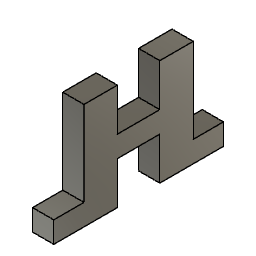
H shape (Autodesk Fusion 360 design; units mm, degrees)
Autodesk Fusion 360 part; units mm, degrees
sketch "Sketch1" plane through (0, 0, 0) normal (1, 0, 0) x (0, 1, 0)
  line L0 (0, -5.7569) -> (0, 10)
  line L1 (0, 10) -> (14.2431, 10)
  line L2 (14.2431, 10) -> (14.2431, 50)
  line L3 (14.2431, 50) -> (30, 50)
  line L4 (30, 30) -> (50, 30)
  line L5 (50, 30) -> (50, 50)
  line L6 (50, 50) -> (65.7569, 50)
  line L7 (25, -25) -> (23.7742, -25.0601)
  line L8 (65.7569, 50) -> (65.7569, 10)
  line L9 (65.7569, 10) -> (80, 10)
  line L10 (80, 10) -> (80, 0)
  line L11 (0, -5.7569) -> (0, 0)
  line L12 (30, 50) -> (30, 30)
  line L13 (30, 20) -> (50, 20)
  line L14 (50, 20) -> (50, 0)
  line L15 (30, 20) -> (30, 0)
  line L16 (80, 0) -> (50, 0)
  line L17 (30, 0) -> (0, 0)
  dimension "d1" = 10
  dimension "d2" = 80
  dimension "d3" = 20
  dimension "d4" = 15.7569
  dimension "d5" = 50
  dimension "d6" = 10
  dimension "d7" = 30
  constraint vertical L0
  constraint perpendicular L0 L1
  constraint perpendicular L1 L2
  constraint perpendicular L2 L3
  constraint perpendicular L2 L4
  constraint perpendicular L4 L5
  constraint perpendicular L5 L6
  constraint perpendicular L6 L8
  constraint perpendicular L5 L9
  constraint perpendicular L9 L10
  constraint perpendicular L10 L16
  constraint perpendicular L11 L16
  constraint perpendicular L3 L12
  constraint horizontal L13
  constraint perpendicular L14 L16
  constraint coincident L15.end L16
  constraint perpendicular L15 L16
  constraint collinear L16 L17
  constraint collinear L1 L9
  constraint equal L3 L6
  constraint equal L0 L3
  constraint equal L4 L13
  constraint collinear L12 L15
  constraint equal L1 L9
  constraint coincident L11.end L17.end
  constraint collinear L3 L6
  measures "d1" distance of L0.end L11.end
  measures "d2" distance of L10.end L11.end
  measures "d3" distance of L13.start L13.end
  measures "d4" distance of L2.end L3.end
  measures "d5" vertical distance of L6.end L10.end
  measures "d6" distance of L4.start L13.start
  measures "d7" distance of L4.end L14.end
extrude "Extrude1" add sketch "Sketch1" along normal blind 10
